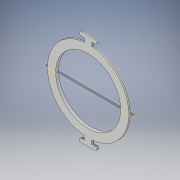
# Autodesk Inventor part: Baseplate_mitte
Saved by Autodesk Inventor 2018 (Build 220112000, 112)
## iProperties
Created: 2020-01-15
Part Number: Baseplate_mitte
Material: Generisch
Document SubType Name: Modeling
Designer: maxse
Density: 1 g/cm^3
Appearance: Vorgabe
Author: maxse
Autodesk Inventor part; units mm, degrees
(part 1 of 3)
ref_plane "YZ Plane" through (0, 0, 0) normal (1, 0, 0) x (0, 1, 0)
ref_plane "XZ Plane" through (0, 0, 0) normal (0, 1, 0) x (-1, 0, 0)
ref_plane "XY Plane" through (0, 0, 0) normal (0, 0, 1) x (1, 0, 0)
sketch "Skizze1" plane through (0, 0, 0) normal (0, 1, 0) x (-1, 0, 0)
  circle A0 centre (0, 0) radius 55
  circle A1 centre (0, 0) radius 44
  line L0 (-9.5, -65) -> (9.5, -65)
  line L1 (-9.5, -60) -> (-5, -60)
  line L2 (-5, -60) -> (-5, -54.7723)
  line L3 (5, -54.7723) -> (5, -60)
  line L4 (5, -60) -> (9.5, -60)
  arc A2 (9.5, -65) -> (9.5, -60) centre (9.5, -62.5) ccw
  arc A3 (-9.5, -60) -> (-9.5, -65) centre (-9.5, -62.5) ccw
  dimension "d0" = 110
  dimension "d1" = 88
  dimension "d2" = 10
  dimension "d3" = 2.5
  dimension "d4" = 2.5
  dimension "d5" = 5
  dimension "d6" = 5
  dimension "d7" = 24
  dimension "d8" = 60
  dimension "d9" = 4.5
  constraints: 10 end point, 6 point on circle, 4 centre point, 2 coincident, 2 horizontal, 2 point on line, 1 parallel, 1 perpendicular
  measures "d0" diameter of A0
  measures "d1" diameter of A1
  measures "d2" distance between parallel lines of L3 L2
  measures "d3" radius of A2
  measures "d4" radius of A3
  measures "d5" distance between parallel lines of L1 L0
  measures "d6" distance from line of point (0, 0) L2
  measures "d8" distance from line of A0.centre L4
  measures "d9" distance from line of L3 A2.centre
extrude "Extrusion1" add sketch "Skizze1" along normal blind 4
mirror "Spiegeln1" about plane through (0, 0, 0) normal (0, 0, 1) of "Extrusion1"
sketch "Skizze2" plane through (0, 4, 0) normal (0, 1, 0) x (1, 0, 0)
  circle A0 centre (0, 0) radius 45 projected
  line L0 (42.831, 23.1383) -> (42.0944, 24.3949)
  line L1 (42.0944, 24.3949) -> (40.8378, 23.6583)
  line L2 (40.8378, 23.6583) -> (40.5946, 24.0731)
  line L3 (40.5946, 24.0731) -> (41.8512, 24.8097)
  line L4 (41.8512, 24.8097) -> (41.1146, 26.0663)
  line L5 (41.1146, 26.0663) -> (41.5144, 26.3007)
  line L6 (41.5144, 26.3007) -> (42.251, 25.0441)
  line L7 (42.251, 25.0441) -> (43.5076, 25.7807)
  line L8 (43.5076, 25.7807) -> (43.7508, 25.3659)
  line L9 (43.7508, 25.3659) -> (42.4942, 24.6293)
  line L10 (42.4942, 24.6293) -> (43.2308, 23.3727)
  line L11 (43.2308, 23.3727) -> (42.831, 23.1383)
  line L12 (44.766, 19.128) -> (44.1473, 20.4466)
  line L13 (44.1473, 20.4466) -> (42.8287, 19.8279)
  line L14 (42.8287, 19.8279) -> (42.6244, 20.2632)
  line L15 (42.6244, 20.2632) -> (43.943, 20.8819)
  line L16 (43.943, 20.8819) -> (43.3243, 22.2006)
  line L17 (43.3243, 22.2006) -> (43.7439, 22.3974)
  line L18 (43.7439, 22.3974) -> (44.3626, 21.0788)
  line L19 (44.3626, 21.0788) -> (45.6812, 21.6975)
  line L20 (45.6812, 21.6975) -> (45.8855, 21.2622)
  line L21 (45.8855, 21.2622) -> (44.5669, 20.6435)
  line L22 (44.5669, 20.6435) -> (45.1856, 19.3248)
  line L23 (45.1856, 19.3248) -> (44.766, 19.128)
  line L24 (46.3265, 14.9576) -> (45.8309, 16.3272)
  line L25 (45.8309, 16.3272) -> (44.4612, 15.8316)
  line L26 (44.4612, 15.8316) -> (44.2976, 16.2838)
  line L27 (44.2976, 16.2838) -> (45.6672, 16.7794)
  line L28 (45.6672, 16.7794) -> (45.1716, 18.1491)
  line L29 (45.1716, 18.1491) -> (45.6074, 18.3068)
  line L30 (45.6074, 18.3068) -> (46.103, 16.9371)
  line L31 (46.103, 16.9371) -> (47.4727, 17.4328)
  line L32 (47.4727, 17.4328) -> (47.6363, 16.9806)
  line L33 (47.6363, 16.9806) -> (46.2667, 16.4849)
  line L34 (46.2667, 16.4849) -> (46.7623, 15.1153)
  line L35 (46.7623, 15.1153) -> (46.3265, 14.9576)
  line L36 (48.9055, 8.9669) -> (48.7236, 9.7939)
  line L37 (48.7236, 9.7939) -> (47.6091, 9.8164)
  line L38 (47.6091, 9.8164) -> (47.7745, 9.0643)
  line L39 (47.7745, 9.0643) -> (47.3933, 8.9805)
  line L40 (47.3933, 8.9805) -> (47.2062, 9.8313)
  line L41 (47.2062, 9.8313) -> (45.9534, 9.8662)
  line L42 (45.9534, 9.8662) -> (45.8733, 10.2304)
  line L43 (45.8733, 10.2304) -> (47.1262, 10.1954)
  line L44 (47.1262, 10.1954) -> (46.957, 10.9646)
  line L45 (46.957, 10.9646) -> (45.7042, 10.9995)
  line L46 (45.7042, 10.9995) -> (45.6241, 11.3637)
  line L47 (45.6241, 11.3637) -> (46.877, 11.3287)
  line L48 (46.877, 11.3287) -> (46.7168, 12.0571)
  line L49 (46.7168, 12.0571) -> (47.098, 12.1409)
  line L50 (47.098, 12.1409) -> (47.2798, 11.3139)
  line L51 (47.2798, 11.3139) -> (48.3944, 11.2913)
  line L52 (48.3944, 11.2913) -> (48.229, 12.0434)
  line L53 (48.229, 12.0434) -> (48.6102, 12.1273)
  line L54 (48.6102, 12.1273) -> (48.7973, 11.2764)
  line L55 (48.7973, 11.2764) -> (50.0535, 11.2422)
  line L56 (50.0535, 11.2422) -> (50.1336, 10.8781)
  line L57 (50.1336, 10.8781) -> (48.8773, 10.9123)
  line L58 (48.8773, 10.9123) -> (49.0464, 10.1431)
  line L59 (49.0464, 10.1431) -> (50.3027, 10.1089)
  line L60 (50.3027, 10.1089) -> (50.3828, 9.7448)
  line L61 (50.3828, 9.7448) -> (49.1265, 9.779)
  line L62 (49.1265, 9.779) -> (49.2866, 9.0507)
  line L63 (49.2866, 9.0507) -> (48.9055, 8.9669)
  line L64 (48.6526, 10.1493) -> (48.4813, 10.9287)
  line L65 (48.4813, 10.9287) -> (47.3516, 10.955)
  line L66 (47.3516, 10.955) -> (47.523, 10.1757)
  line L67 (47.523, 10.1757) -> (48.6526, 10.1493)
  spline S0 degree 2 poles (48.4497, 5.1486) (47.6487, 5.0391) (46.5984, 5.6727) (46.5186, 6.2562) knots 0 0 0 1 2 2 2
  spline S1 degree 2 poles (46.5186, 6.2562) (46.486, 6.4944) (46.5464, 6.8755) (46.6344, 7.0809) knots 0 0 0 1 2 2 2
  line L68 (46.6344, 7.0809) -> (45.2948, 6.8977)
  line L69 (45.2948, 6.8977) -> (45.2212, 7.4363)
  line L70 (45.2212, 7.4363) -> (49.5955, 8.0345)
  line L71 (49.5955, 8.0345) -> (49.6691, 7.496)
  line L72 (49.6691, 7.496) -> (49.3342, 7.4502)
  spline S2 degree 2 poles (49.3342, 7.4502) (49.5446, 7.2749) (49.8533, 6.8177) (49.8925, 6.5312) knots 0 0 0 1 2 2 2
  spline S3 degree 2 poles (49.8925, 6.5312) (49.9676, 5.9822) (49.1816, 5.2487) (48.4497, 5.1486) knots 0 0 0 1 2 2 2
  spline S4 degree 2 poles (48.3115, 5.696) (48.8605, 5.771) (49.417, 6.2024) (49.3636, 6.5925) knots 0 0 0 1 2 2 2
  spline S5 degree 2 poles (49.3636, 6.5925) (49.3324, 6.8204) (49.0702, 7.2206) (48.8854, 7.3888) knots 0 0 0 1 2 2 2
  line L73 (48.8854, 7.3888) -> (47.0694, 7.1404)
  spline S6 degree 2 poles (47.0694, 7.1404) (46.9981, 6.9161) (46.9632, 6.6054) (46.9897, 6.412) knots 0 0 0 1 2 2 2
  spline S7 degree 2 poles (46.9897, 6.412) (47.0468, 5.9943) (47.7246, 5.6157) (48.3115, 5.696) knots 0 0 0 1 2 2 2
  line L74 (46.8467, 3.8024) -> (46.7996, 4.344)
  line L75 (46.7996, 4.344) -> (50.0142, 4.6236)
  line L76 (50.0142, 4.6236) -> (50.0613, 4.0821)
  line L77 (50.0613, 4.0821) -> (46.8467, 3.8024)
  line L78 (50.5993, 4.0904) -> (50.5458, 4.7048)
  line L79 (50.5458, 4.7048) -> (51.1082, 4.7538)
  line L80 (51.1082, 4.7538) -> (51.1616, 4.1393)
  line L81 (51.1616, 4.1393) -> (50.5993, 4.0904)
  line L82 (47.0217, -0.6477) -> (48.8891, -0.6111)
  spline S8 degree 2 poles (48.8891, -0.6111) (49.1121, -0.6067) (49.4912, -0.5644) (49.5946, -0.5066) knots 0 0 0 1 2 2 2
  spline S9 degree 2 poles (49.5946, -0.5066) (49.7085, -0.4486) (49.8158, -0.2339) (49.8122, -0.0493) knots 0 0 0 1 2 2 2
  spline S10 degree 2 poles (49.8122, -0.0493) (49.8089, 0.118) (49.5958, 0.4972) (49.3968, 0.6954) knots 0 0 0 1 2 2 2
  spline S11 degree 2 poles (49.3968, 0.6954) (49.348, 0.691) (49.2123, 0.6813) (49.1217, 0.6796) knots 0 0 0 1 2 2 2
  line L83 (49.1217, 0.6796) -> (46.9965, 0.6379)
  line L84 (46.9965, 0.6379) -> (46.9859, 1.1814)
  line L85 (46.9859, 1.1814) -> (48.8533, 1.218)
  spline S12 degree 2 poles (48.8533, 1.218) (49.0762, 1.2224) (49.4553, 1.2647) (49.5587, 1.3225) knots 0 0 0 1 2 2 2
  spline S13 degree 2 poles (49.5587, 1.3225) (49.6726, 1.3805) (49.7799, 1.5952) (49.7763, 1.7798) knots 0 0 0 1 2 2 2
  spline S14 degree 2 poles (49.7763, 1.7798) (49.7729, 1.954) (49.5458, 2.3364) (49.3715, 2.5142) knots 0 0 0 1 2 2 2
  line L86 (49.3715, 2.5142) -> (46.9606, 2.4669)
  line L87 (46.9606, 2.4669) -> (46.95, 3.0104)
  line L88 (46.95, 3.0104) -> (50.1761, 3.0737)
  line L89 (50.1761, 3.0737) -> (50.1868, 2.5302)
  line L90 (50.1868, 2.5302) -> (49.8314, 2.5233)
  spline S15 degree 2 poles (49.8314, 2.5233) (50.0481, 2.3149) (50.2897, 1.9014) (50.2946, 1.6506) knots 0 0 0 1 2 2 2
  spline S16 degree 2 poles (50.2946, 1.6506) (50.3002, 1.3649) (50.0476, 0.9173) (49.7538, 0.7965) knots 0 0 0 1 2 2 2
  spline S17 degree 2 poles (49.7538, 0.7965) (50.0338, 0.5546) (50.3252, 0.0933) (50.3305, -0.1785) knots 0 0 0 1 2 2 2
  spline S18 degree 2 poles (50.3305, -0.1785) (50.3346, -0.3875) (50.2124, -0.7315) (50.0686, -0.8598) knots 0 0 0 1 2 2 2
  spline S19 degree 2 poles (50.0686, -0.8598) (49.9248, -0.9916) (49.4886, -1.143) (49.1576, -1.1495) knots 0 0 0 1 2 2 2
  line L91 (49.1576, -1.1495) -> (47.0324, -1.1912)
  line L92 (47.0324, -1.1912) -> (47.0217, -0.6477)
  spline S20 degree 2 poles (48.4889, -4.7653) (47.6823, -4.7105) (46.782, -3.8773) (46.822, -3.2898) knots 0 0 0 1 2 2 2
  spline S21 degree 2 poles (46.822, -3.2898) (46.8383, -3.0499) (46.9746, -2.689) (47.1023, -2.5056) knots 0 0 0 1 2 2 2
  line L93 (47.1023, -2.5056) -> (45.7534, -2.4138)
  line L94 (45.7534, -2.4138) -> (45.7903, -1.8715)
  line L95 (45.7903, -1.8715) -> (50.1951, -2.1711)
  line L96 (50.1951, -2.1711) -> (50.1582, -2.7134)
  line L97 (50.1582, -2.7134) -> (49.821, -2.6905)
  spline S22 degree 2 poles (49.821, -2.6905) (49.9916, -2.9047) (50.2013, -3.4149) (50.1817, -3.7035) knots 0 0 0 1 2 2 2
  spline S23 degree 2 poles (50.1817, -3.7035) (50.1441, -4.2562) (49.2259, -4.8155) (48.4889, -4.7653) knots 0 0 0 1 2 2 2
  spline S24 degree 2 poles (48.4644, -4.2013) (49.0171, -4.2389) (49.6494, -3.9292) (49.6762, -3.5363) knots 0 0 0 1 2 2 2
  spline S25 degree 2 poles (49.6762, -3.5363) (49.6918, -3.3069) (49.516, -2.8618) (49.3691, -2.6598) knots 0 0 0 1 2 2 2
  line L98 (49.3691, -2.6598) -> (47.5404, -2.5354)
  spline S26 degree 2 poles (47.5404, -2.5354) (47.4251, -2.7406) (47.3281, -3.0378) (47.3148, -3.2325) knots 0 0 0 1 2 2 2
  spline S27 degree 2 poles (47.3148, -3.2325) (47.2862, -3.6532) (47.8734, -4.1611) (48.4644, -4.2013) knots 0 0 0 1 2 2 2
  line L99 (49.5822, -8.1516) -> (45.4386, -5.842)
  line L100 (45.4386, -5.842) -> (45.5163, -5.2653)
  line L101 (45.5163, -5.2653) -> (46.7721, -6.0183)
  line L102 (46.7721, -6.0183) -> (49.9709, -5.2681)
  line L103 (49.9709, -5.2681) -> (49.8927, -5.8482)
  line L104 (49.8927, -5.8482) -> (47.4059, -6.4026)
  line L105 (47.4059, -6.4026) -> (49.6576, -7.5922)
  line L106 (49.6576, -7.5922) -> (49.5822, -8.1516)
  spline S28 degree 2 poles (47.3643, -11.0433) (46.5651, -10.8818) (45.8495, -9.9373) (45.9793, -9.2951) knots 0 0 0 1 2 2 2
  spline S29 degree 2 poles (45.9793, -9.2951) (46.1125, -8.6359) (47.1633, -8.0627) (47.9353, -8.2187) knots 0 0 0 1 2 2 2
  spline S30 degree 2 poles (47.9353, -8.2187) (48.7277, -8.3789) (49.4481, -9.335) (49.3196, -9.9703) knots 0 0 0 1 2 2 2
  spline S31 degree 2 poles (49.3196, -9.9703) (49.1899, -10.6124) (48.1602, -11.2042) (47.3643, -11.0433) knots 0 0 0 1 2 2 2
  spline S32 degree 2 poles (47.4755, -10.4934) (48.0903, -10.6177) (48.7784, -10.2911) (48.862, -9.8778) knots 0 0 0 1 2 2 2
  spline S33 degree 2 poles (48.862, -9.8778) (48.9455, -9.4645) (48.4389, -8.8929) (47.8241, -8.7686) knots 0 0 0 1 2 2 2
  spline S34 degree 2 poles (47.8241, -8.7686) (47.2264, -8.6478) (46.5205, -8.9744) (46.4369, -9.3877) knots 0 0 0 1 2 2 2
  spline S35 degree 2 poles (46.4369, -9.3877) (46.3541, -9.7975) (46.8675, -10.3706) (47.4755, -10.4934) knots 0 0 0 1 2 2 2
  line L107 (44.9816, -13.6832) -> (45.1259, -13.1591)
  line L108 (45.1259, -13.1591) -> (45.4686, -13.2534)
  spline S36 degree 2 poles (45.4686, -13.2534) (45.3235, -12.9532) (45.2244, -12.4597) (45.2984, -12.191) knots 0 0 0 1 2 2 2
  spline S37 degree 2 poles (45.2984, -12.191) (45.3539, -11.9894) (45.5872, -11.6669) (45.7678, -11.5756) knots 0 0 0 1 2 2 2
  spline S38 degree 2 poles (45.7678, -11.5756) (45.9492, -11.481) (46.43, -11.4543) (46.7458, -11.5413) knots 0 0 0 1 2 2 2
  line L109 (46.7458, -11.5413) -> (48.765, -12.0971)
  line L110 (48.765, -12.0971) -> (48.6207, -12.6212)
  line L111 (48.6207, -12.6212) -> (46.8468, -12.1329)
  spline S39 degree 2 poles (46.8468, -12.1329) (46.5982, -12.0645) (46.2621, -12.0117) (46.1236, -12.0422) knots 0 0 0 1 2 2 2
  spline S40 degree 2 poles (46.1236, -12.0422) (45.9851, -12.0728) (45.8141, -12.2606) (45.7577, -12.4656) knots 0 0 0 1 2 2 2
  spline S41 degree 2 poles (45.7577, -12.4656) (45.705, -12.6571) (45.8041, -13.1506) (45.912, -13.3755) knots 0 0 0 1 2 2 2
  line L112 (45.912, -13.3755) -> (48.2369, -14.0154)
  line L113 (48.2369, -14.0154) -> (48.0926, -14.5395)
  line L114 (48.0926, -14.5395) -> (44.9816, -13.6832)
  line L115 (46.6915, -16.8993) -> (46.7005, -16.8729)
  spline S42 degree 2 poles (46.7005, -16.8729) (46.7371, -16.8191) (46.7873, -16.6926) (46.8174, -16.6035) knots 0 0 0 1 2 2 2
  spline S43 degree 2 poles (46.8174, -16.6035) (46.8878, -16.3955) (46.8448, -15.9248) (46.7291, -15.6796) knots 0 0 0 1 2 2 2
  line L116 (46.7291, -15.6796) -> (44.5606, -14.9457)
  line L117 (44.5606, -14.9457) -> (44.7348, -14.4308)
  line L118 (44.7348, -14.4308) -> (47.7913, -15.4652)
  line L119 (47.7913, -15.4652) -> (47.617, -15.9801)
  line L120 (47.617, -15.9801) -> (47.1615, -15.826)
  spline S44 degree 2 poles (47.1615, -15.826) (47.3174, -16.1914) (47.3802, -16.6799) (47.3131, -16.8779) knots 0 0 0 1 2 2 2
  spline S45 degree 2 poles (47.3131, -16.8779) (47.2863, -16.9571) (47.2529, -17.0341) (47.2262, -17.0803) knots 0 0 0 1 2 2 2
  line L121 (47.2262, -17.0803) -> (46.6915, -16.8993)
  spline S46 degree 2 poles (44.6095, -19.5926) (43.8599, -19.2899) (43.263, -18.2183) (43.4835, -17.6722) knots 0 0 0 1 2 2 2
  spline S47 degree 2 poles (43.4835, -17.6722) (43.5735, -17.4493) (43.8152, -17.1485) (43.9936, -17.0139) knots 0 0 0 1 2 2 2
  line L122 (43.9936, -17.0139) -> (42.7399, -16.5076)
  line L123 (42.7399, -16.5076) -> (42.9435, -16.0036)
  line L124 (42.9435, -16.0036) -> (47.0373, -17.6567)
  line L125 (47.0373, -17.6567) -> (46.8337, -18.1608)
  line L126 (46.8337, -18.1608) -> (46.5203, -18.0342)
  spline S48 degree 2 poles (46.5203, -18.0342) (46.6159, -18.2908) (46.6568, -18.8409) (46.5485, -19.1091) knots 0 0 0 1 2 2 2
  spline S49 degree 2 poles (46.5485, -19.1091) (46.341, -19.6228) (45.2945, -19.8692) (44.6095, -19.5926) knots 0 0 0 1 2 2 2
  spline S50 degree 2 poles (44.7614, -19.0489) (45.2752, -19.2563) (45.9724, -19.1583) (46.1199, -18.7932) knots 0 0 0 1 2 2 2
  spline S51 degree 2 poles (46.1199, -18.7932) (46.206, -18.58) (46.1771, -18.1023) (46.1003, -17.8646) knots 0 0 0 1 2 2 2
  line L127 (46.1003, -17.8646) -> (44.4007, -17.1783)
  spline S52 degree 2 poles (44.4007, -17.1783) (44.2274, -17.3375) (44.0428, -17.5899) (43.9697, -17.7709) knots 0 0 0 1 2 2 2
  spline S53 degree 2 poles (43.9697, -17.7709) (43.8119, -18.1618) (44.2122, -18.8271) (44.7614, -19.0489) knots 0 0 0 1 2 2 2
  line L128 (44.4466, -22.1401) -> (44.4585, -22.1149)
  spline S54 degree 2 poles (44.4585, -22.1149) (44.501, -22.0657) (44.5654, -21.9457) (44.6056, -21.8607) knots 0 0 0 1 2 2 2
  spline S55 degree 2 poles (44.6056, -21.8607) (44.6993, -21.6622) (44.7105, -21.1896) (44.6237, -20.9328) knots 0 0 0 1 2 2 2
  line L129 (44.6237, -20.9328) -> (42.5536, -19.9551)
  line L130 (42.5536, -19.9551) -> (42.7858, -19.4636)
  line L131 (42.7858, -19.4636) -> (45.7035, -20.8416)
  line L132 (45.7035, -20.8416) -> (45.4713, -21.3331)
  line L133 (45.4713, -21.3331) -> (45.0365, -21.1277)
  spline S56 degree 2 poles (45.0365, -21.1277) (45.1495, -21.5087) (45.1558, -22.0011) (45.0665, -22.1901) knots 0 0 0 1 2 2 2
  spline S57 degree 2 poles (45.0665, -22.1901) (45.0308, -22.2658) (44.9888, -22.3384) (44.957, -22.3812) knots 0 0 0 1 2 2 2
  line L134 (44.957, -22.3812) -> (44.4466, -22.1401)
  line L135 (41.6005, -21.8741) -> (41.8507, -21.3915)
  line L136 (41.8507, -21.3915) -> (44.7153, -22.8766)
  line L137 (44.7153, -22.8766) -> (44.4651, -23.3592)
  line L138 (44.4651, -23.3592) -> (41.6005, -21.8741)
  line L139 (44.9239, -23.6403) -> (45.2078, -23.0927)
  line L140 (45.2078, -23.0927) -> (45.7089, -23.3525)
  line L141 (45.7089, -23.3525) -> (45.425, -23.9001)
  line L142 (45.425, -23.9001) -> (44.9239, -23.6403)
  line L143 (39.9616, -24.7731) -> (40.2353, -24.3035)
  line L144 (40.2353, -24.3035) -> (41.8249, -25.23)
  spline S58 degree 2 poles (41.8249, -25.23) (42.0176, -25.3423) (42.3698, -25.4992) (42.5007, -25.5029) knots 0 0 0 1 2 2 2
  spline S59 degree 2 poles (42.5007, -25.5029) (42.6394, -25.5071) (42.8611, -25.3621) (42.9629, -25.1875) knots 0 0 0 1 2 2 2
  spline S60 degree 2 poles (42.9629, -25.1875) (43.0646, -25.0129) (43.0938, -24.5338) (43.0468, -24.2684) knots 0 0 0 1 2 2 2
  line L145 (43.0468, -24.2684) -> (40.9636, -23.0541)
  line L146 (40.9636, -23.0541) -> (41.2373, -22.5845)
  line L147 (41.2373, -22.5845) -> (44.025, -24.2094)
  line L148 (44.025, -24.2094) -> (43.7513, -24.679)
  line L149 (43.7513, -24.679) -> (43.4412, -24.4983)
  spline S61 degree 2 poles (43.4412, -24.4983) (43.508, -24.8196) (43.4698, -25.3418) (43.3365, -25.5706) knots 0 0 0 1 2 2 2
  spline S62 degree 2 poles (43.3365, -25.5706) (43.0978, -25.98) (42.2857, -26.1278) (41.7709, -25.8277) knots 0 0 0 1 2 2 2
  line L150 (41.7709, -25.8277) -> (39.9616, -24.7731)
  spline S63 degree 2 poles (38.9527, -26.1904) (39.1967, -25.8212) (39.8929, -25.6839) (40.3494, -25.9855) knots 0 0 0 1 2 2 2
  line L151 (40.3494, -25.9855) -> (41.8409, -26.9709)
  line L152 (41.8409, -26.9709) -> (42.0426, -26.6656)
  line L153 (42.0426, -26.6656) -> (42.4176, -26.9134)
  line L154 (42.4176, -26.9134) -> (42.2159, -27.2187)
  line L155 (42.2159, -27.2187) -> (42.9893, -27.7296)
  line L156 (42.9893, -27.7296) -> (42.6896, -28.1832)
  line L157 (42.6896, -28.1832) -> (41.9163, -27.6722)
  line L158 (41.9163, -27.6722) -> (41.365, -28.5066)
  line L159 (41.365, -28.5066) -> (40.9899, -28.2589)
  line L160 (40.9899, -28.2589) -> (41.5412, -27.4244)
  line L161 (41.5412, -27.4244) -> (40.2591, -26.5774)
  spline S64 degree 2 poles (40.2591, -26.5774) (40.0555, -26.4429) (39.8221, -26.3095) (39.6935, -26.2956) knots 0 0 0 1 2 2 2
  spline S65 degree 2 poles (39.6935, -26.2956) (39.5823, -26.2806) (39.3769, -26.408) (39.2732, -26.565) knots 0 0 0 1 2 2 2
  spline S66 degree 2 poles (39.2732, -26.565) (39.2002, -26.6755) (39.1307, -26.9261) (39.1203, -26.9861) knots 0 0 0 1 2 2 2
  line L162 (39.1203, -26.9861) -> (39.1031, -27.0122)
  line L163 (39.1031, -27.0122) -> (38.696, -26.7433)
  spline S67 degree 2 poles (38.696, -26.7433) (38.7456, -26.5923) (38.8778, -26.3038) (38.9527, -26.1904) knots 0 0 0 1 2 2 2
  line L164 (36.4432, -32.2764) -> (37.3703, -31.153)
  line L165 (37.3703, -31.153) -> (36.2468, -30.2259)
  line L166 (36.2468, -30.2259) -> (36.5529, -29.855)
  line L167 (36.5529, -29.855) -> (37.6763, -30.7821)
  line L168 (37.6763, -30.7821) -> (38.6034, -29.6587)
  line L169 (38.6034, -29.6587) -> (38.9609, -29.9537)
  line L170 (38.9609, -29.9537) -> (38.0338, -31.0771)
  line L171 (38.0338, -31.0771) -> (39.1572, -32.0042)
  line L172 (39.1572, -32.0042) -> (38.8511, -32.3751)
  line L173 (38.8511, -32.3751) -> (37.7277, -31.448)
  line L174 (37.7277, -31.448) -> (36.8006, -32.5714)
  line L175 (36.8006, -32.5714) -> (36.4432, -32.2764)
  line L176 (33.3416, -35.4713) -> (34.3674, -34.4373)
  line L177 (34.3674, -34.4373) -> (33.3334, -33.4114)
  line L178 (33.3334, -33.4114) -> (33.6721, -33.0701)
  line L179 (33.6721, -33.0701) -> (34.7061, -34.0959)
  line L180 (34.7061, -34.0959) -> (35.732, -33.0619)
  line L181 (35.732, -33.0619) -> (36.061, -33.3883)
  line L182 (36.061, -33.3883) -> (35.0351, -34.4223)
  line L183 (35.0351, -34.4223) -> (36.0691, -35.4482)
  line L184 (36.0691, -35.4482) -> (35.7304, -35.7896)
  line L185 (35.7304, -35.7896) -> (34.6964, -34.7637)
  line L186 (34.6964, -34.7637) -> (33.6706, -35.7977)
  line L187 (33.6706, -35.7977) -> (33.3416, -35.4713)
  line L188 (29.961, -38.3694) -> (31.077, -37.4335)
  line L189 (31.077, -37.4335) -> (30.1411, -36.3174)
  line L190 (30.1411, -36.3174) -> (30.5095, -36.0084)
  line L191 (30.5095, -36.0084) -> (31.4455, -37.1245)
  line L192 (31.4455, -37.1245) -> (32.5616, -36.1885)
  line L193 (32.5616, -36.1885) -> (32.8594, -36.5436)
  line L194 (32.8594, -36.5436) -> (31.7433, -37.4796)
  line L195 (31.7433, -37.4796) -> (32.6793, -38.5956)
  line L196 (32.6793, -38.5956) -> (32.3108, -38.9046)
  line L197 (32.3108, -38.9046) -> (31.3749, -37.7886)
  line L198 (31.3749, -37.7886) -> (30.2588, -38.7245)
  line L199 (30.2588, -38.7245) -> (29.961, -38.3694)
  line L200 (23.5821, -40.6975) -> (24.065, -40.3918)
  line L201 (24.065, -40.3918) -> (26.0462, -43.5215)
  line L202 (26.0462, -43.5215) -> (25.6467, -40.7927)
  line L203 (25.6467, -40.7927) -> (25.9411, -40.6063)
  line L204 (25.9411, -40.6063) -> (28.2279, -42.1404)
  line L205 (28.2279, -42.1404) -> (26.2466, -39.0107)
  line L206 (26.2466, -39.0107) -> (26.6971, -38.7255)
  line L207 (26.6971, -38.7255) -> (28.9971, -42.3587)
  line L208 (28.9971, -42.3587) -> (28.3376, -42.7762)
  line L209 (28.3376, -42.7762) -> (26.1503, -41.3276)
  line L210 (26.1503, -41.3276) -> (26.5534, -43.9057)
  line L211 (26.5534, -43.9057) -> (25.8821, -44.3306)
  line L212 (25.8821, -44.3306) -> (23.5821, -40.6975)
  spline S68 degree 2 poles (21.5761, -41.6732) (22.2613, -41.314) (23.4172, -41.6877) (23.7893, -42.3976) knots 0 0 0 1 2 2 2
  spline S69 degree 2 poles (23.7893, -42.3976) (24.1549, -43.0951) (23.8571, -44.3056) (23.2676, -44.6146) knots 0 0 0 1 2 2 2
  spline S70 degree 2 poles (23.2676, -44.6146) (23.0022, -44.7538) (22.5108, -44.8146) (22.2738, -44.7303) knots 0 0 0 1 2 2 2
  spline S71 degree 2 poles (22.2738, -44.7303) (22.0338, -44.6477) (21.6227, -44.2612) (21.4431, -43.9186) knots 0 0 0 1 2 2 2
  line L213 (21.4431, -43.9186) -> (21.3056, -43.6563)
  line L214 (21.3056, -43.6563) -> (23.2839, -42.6193)
  spline S72 degree 2 poles (23.2839, -42.6193) (23.0234, -42.1224) (22.2468, -41.8567) (21.8023, -42.0897) knots 0 0 0 1 2 2 2
  spline S73 degree 2 poles (21.8023, -42.0897) (21.6449, -42.1722) (21.3766, -42.4033) (21.2823, -42.5236) knots 0 0 0 1 2 2 2
  spline S74 degree 2 poles (21.2823, -42.5236) (21.185, -42.6533) (21.0626, -42.8551) (21.0299, -42.9353) knots 0 0 0 1 2 2 2
  line L215 (21.0299, -42.9353) -> (21.0021, -42.9498)
  line L216 (21.0021, -42.9498) -> (20.7271, -42.4252)
  spline S75 degree 2 poles (20.7271, -42.4252) (20.7926, -42.3475) (20.9939, -42.1161) (21.0781, -42.0366) knots 0 0 0 1 2 2 2
  spline S76 degree 2 poles (21.0781, -42.0366) (21.1959, -41.9236) (21.4033, -41.7638) (21.5761, -41.6732) knots 0 0 0 1 2 2 2
  spline S77 degree 2 poles (21.9672, -43.7777) (22.0753, -43.9688) (22.3044, -44.2107) (22.4317, -44.2659) knots 0 0 0 1 2 2 2
  spline S78 degree 2 poles (22.4317, -44.2659) (22.5716, -44.3303) (22.8938, -44.307) (23.0883, -44.205) knots 0 0 0 1 2 2 2
  spline S79 degree 2 poles (23.0883, -44.205) (23.2796, -44.1047) (23.4883, -43.8498) (23.5411, -43.6804) knots 0 0 0 1 2 2 2
  spline S80 degree 2 poles (23.5411, -43.6804) (23.5893, -43.5096) (23.5564, -43.1767) (23.4764, -42.9865) knots 0 0 0 1 2 2 2
  line L217 (23.4764, -42.9865) -> (21.9672, -43.7777)
  line L218 (16.7233, -43.9522) -> (17.4454, -45.6747)
  spline S81 degree 2 poles (17.4454, -45.6747) (17.5317, -45.8804) (17.7106, -46.2172) (17.8025, -46.292) knots 0 0 0 1 2 2 2
  spline S82 degree 2 poles (17.8025, -46.292) (17.8984, -46.3765) (18.1375, -46.3972) (18.3078, -46.3258) knots 0 0 0 1 2 2 2
  spline S83 degree 2 poles (18.3078, -46.3258) (18.4621, -46.2611) (18.7361, -45.9233) (18.847, -45.6652) knots 0 0 0 1 2 2 2
  spline S84 degree 2 poles (18.847, -45.6652) (18.825, -45.6216) (18.766, -45.4989) (18.731, -45.4154) knots 0 0 0 1 2 2 2
  line L219 (18.731, -45.4154) -> (17.9092, -43.4551)
  line L220 (17.9092, -43.4551) -> (18.4105, -43.2449)
  line L221 (18.4105, -43.2449) -> (19.1326, -44.9674)
  spline S85 degree 2 poles (19.1326, -44.9674) (19.2188, -45.1731) (19.3978, -45.5099) (19.4896, -45.5847) knots 0 0 0 1 2 2 2
  spline S86 degree 2 poles (19.4896, -45.5847) (19.5855, -45.6692) (19.8247, -45.6899) (19.995, -45.6185) knots 0 0 0 1 2 2 2
  spline S87 degree 2 poles (19.995, -45.6185) (20.1557, -45.5511) (20.4275, -45.1991) (20.5286, -44.9716) knots 0 0 0 1 2 2 2
  line L222 (20.5286, -44.9716) -> (19.5963, -42.7478)
  line L223 (19.5963, -42.7478) -> (20.0977, -42.5376)
  line L224 (20.0977, -42.5376) -> (21.3452, -45.5134)
  line L225 (21.3452, -45.5134) -> (20.8438, -45.7236)
  line L226 (20.8438, -45.7236) -> (20.7064, -45.3958)
  spline S88 degree 2 poles (20.7064, -45.3958) (20.5926, -45.674) (20.2972, -46.051) (20.0658, -46.148) knots 0 0 0 1 2 2 2
  spline S89 degree 2 poles (20.0658, -46.148) (19.8023, -46.2585) (19.2931, -46.1885) (19.0726, -45.9598) knots 0 0 0 1 2 2 2
  spline S90 degree 2 poles (19.0726, -45.9598) (18.9508, -46.3094) (18.6293, -46.7502) (18.3787, -46.8553) knots 0 0 0 1 2 2 2
  spline S91 degree 2 poles (18.3787, -46.8553) (18.1858, -46.9361) (17.8211, -46.9492) (17.6488, -46.8628) knots 0 0 0 1 2 2 2
  spline S92 degree 2 poles (17.6488, -46.8628) (17.4733, -46.7776) (17.1718, -46.428) (17.0438, -46.1227) knots 0 0 0 1 2 2 2
  line L227 (17.0438, -46.1227) -> (16.222, -44.1623)
  line L228 (16.222, -44.1623) -> (16.7233, -43.9522)
  spline S93 degree 2 poles (13.4254, -46.8001) (13.1845, -46.0466) (13.6208, -44.8938) (14.1717, -44.7176) knots 0 0 0 1 2 2 2
  spline S94 degree 2 poles (14.1717, -44.7176) (14.4207, -44.6381) (14.8151, -44.6473) (15.0216, -44.6984) knots 0 0 0 1 2 2 2
  line L229 (15.0216, -44.6984) -> (15.0092, -44.545)
  line L230 (15.0092, -44.545) -> (15.4938, -44.3901)
  line L231 (15.4938, -44.3901) -> (16.8615, -48.6684)
  line L232 (16.8615, -48.6684) -> (16.3438, -48.834)
  line L233 (16.3438, -48.834) -> (15.8557, -47.3072)
  spline S95 degree 2 poles (15.8557, -47.3072) (15.7161, -47.5457) (15.3356, -47.9234) (15.0469, -48.0157) knots 0 0 0 1 2 2 2
  spline S96 degree 2 poles (15.0469, -48.0157) (14.5258, -48.1823) (13.662, -47.5402) (13.4254, -46.8001) knots 0 0 0 1 2 2 2
  spline S97 degree 2 poles (13.947, -46.5894) (14.1231, -47.1404) (14.6409, -47.6041) (15.0126, -47.4852) knots 0 0 0 1 2 2 2
  spline S98 degree 2 poles (15.0126, -47.4852) (15.2217, -47.4184) (15.5895, -47.0813) (15.7166, -46.8724) knots 0 0 0 1 2 2 2
  line L234 (15.7166, -46.8724) -> (15.1532, -45.1099)
  spline S99 degree 2 poles (15.1532, -45.1099) (14.9266, -45.0763) (14.5991, -45.0932) (14.4199, -45.1505) knots 0 0 0 1 2 2 2
  spline S100 degree 2 poles (14.4199, -45.1505) (14.0249, -45.2768) (13.7528, -45.982) (13.947, -46.5894) knots 0 0 0 1 2 2 2
  line L235 (11.3723, -48.3359) -> (11.3993, -48.3289)
  spline S101 degree 2 poles (11.3993, -48.3289) (11.4644, -48.3302) (11.5977, -48.303) (11.6888, -48.2796) knots 0 0 0 1 2 2 2
  spline S102 degree 2 poles (11.6888, -48.2796) (11.9014, -48.2248) (12.2721, -47.9315) (12.4141, -47.7006) knots 0 0 0 1 2 2 2
  line L236 (12.4141, -47.7006) -> (11.8433, -45.4835)
  line L237 (11.8433, -45.4835) -> (12.3698, -45.348)
  line L238 (12.3698, -45.348) -> (13.1743, -48.4728)
  line L239 (13.1743, -48.4728) -> (12.6478, -48.6084)
  line L240 (12.6478, -48.6084) -> (12.528, -48.1427)
  spline S103 degree 2 poles (12.528, -48.1427) (12.3071, -48.473) (11.9324, -48.7926) (11.73, -48.8447) knots 0 0 0 1 2 2 2
  spline S104 degree 2 poles (11.73, -48.8447) (11.649, -48.8655) (11.5663, -48.8796) (11.513, -48.8826) knots 0 0 0 1 2 2 2
  line L241 (11.513, -48.8826) -> (11.3723, -48.3359)
  spline S105 degree 2 poles (8.6058, -46.5571) (8.6612, -46.4964) (8.846, -46.282) (8.9383, -46.2103) knots 0 0 0 1 2 2 2
  spline S106 degree 2 poles (8.9383, -46.2103) (9.0635, -46.1073) (9.311, -45.9763) (9.5503, -45.9288) knots 0 0 0 1 2 2 2
  spline S107 degree 2 poles (9.5503, -45.9288) (9.7451, -45.89) (10.1263, -45.967) (10.2861, -46.0738) knots 0 0 0 1 2 2 2
  spline S108 degree 2 poles (10.2861, -46.0738) (10.4384, -46.1785) (10.6683, -46.5307) (10.7104, -46.7426) knots 0 0 0 1 2 2 2
  spline S109 degree 2 poles (10.7104, -46.7426) (10.7757, -47.0707) (10.5913, -47.5906) (10.317, -47.7837) knots 0 0 0 1 2 2 2
  spline S110 degree 2 poles (10.317, -47.7837) (10.0749, -47.9597) (9.3687, -48.196) (8.9531, -48.3036) knots 0 0 0 1 2 2 2
  line L242 (8.9531, -48.3036) -> (8.9735, -48.4061)
  spline S111 degree 2 poles (8.9735, -48.4061) (9.0102, -48.5906) (9.1685, -48.7972) (9.2839, -48.8418) knots 0 0 0 1 2 2 2
  spline S112 degree 2 poles (9.2839, -48.8418) (9.3994, -48.8863) (9.7014, -48.8689) (9.8587, -48.8376) knots 0 0 0 1 2 2 2
  spline S113 degree 2 poles (9.8587, -48.8376) (10.0432, -48.8009) (10.5204, -48.5923) (10.7489, -48.4368) knots 0 0 0 1 2 2 2
  line L243 (10.7489, -48.4368) -> (10.7796, -48.4306)
  line L244 (10.7796, -48.4306) -> (10.8877, -48.9741)
  spline S114 degree 2 poles (10.8877, -48.9741) (10.7489, -49.0443) (10.219, -49.2562) (9.949, -49.3099) knots 0 0 0 1 2 2 2
  spline S115 degree 2 poles (9.949, -49.3099) (9.6209, -49.3752) (9.1528, -49.3617) (8.9486, -49.2637) knots 0 0 0 1 2 2 2
  spline S116 degree 2 poles (8.9486, -49.2637) (8.7485, -49.1685) (8.4954, -48.7889) (8.4362, -48.4916) knots 0 0 0 1 2 2 2
  line L245 (8.4362, -48.4916) -> (8.006, -46.3282)
  line L246 (8.006, -46.3282) -> (8.5392, -46.2222)
  line L247 (8.5392, -46.2222) -> (8.6058, -46.5571)
  line L248 (8.6942, -47.0014) -> (8.8688, -47.8798)
  spline S117 degree 2 poles (8.8688, -47.8798) (9.0568, -47.8246) (9.6228, -47.6517) (9.7931, -47.561) knots 0 0 0 1 2 2 2
  spline S118 degree 2 poles (9.7931, -47.561) (9.9921, -47.4539) (10.2152, -47.1289) (10.1677, -46.8896) knots 0 0 0 1 2 2 2
  spline S119 degree 2 poles (10.1677, -46.8896) (10.1133, -46.6162) (9.7507, -46.4005) (9.4567, -46.459) knots 0 0 0 1 2 2 2
  spline S120 degree 2 poles (9.4567, -46.459) (9.2072, -46.5086) (8.8399, -46.8055) (8.6942, -47.0014) knots 0 0 0 1 2 2 2
  line L249 (4.7413, -46.7777) -> (5.2804, -46.7082)
  line L250 (5.2804, -46.7082) -> (5.5156, -48.533)
  spline S121 degree 2 poles (5.5156, -48.533) (5.5442, -48.7542) (5.6346, -49.129) (5.7116, -49.235) knots 0 0 0 1 2 2 2
  spline S122 degree 2 poles (5.7116, -49.235) (5.7928, -49.3475) (6.043, -49.4347) (6.2434, -49.4089) knots 0 0 0 1 2 2 2
  spline S123 degree 2 poles (6.2434, -49.4089) (6.4439, -49.383) (6.8413, -49.114) (7.023, -48.9149) knots 0 0 0 1 2 2 2
  line L251 (7.023, -48.9149) -> (6.7146, -46.5233)
  line L252 (6.7146, -46.5233) -> (7.2538, -46.4538)
  line L253 (7.2538, -46.4538) -> (7.6664, -49.6541)
  line L254 (7.6664, -49.6541) -> (7.1272, -49.7236)
  line L255 (7.1272, -49.7236) -> (7.0813, -49.3676)
  spline S124 degree 2 poles (7.0813, -49.3676) (6.8675, -49.6165) (6.4303, -49.9048) (6.1677, -49.9386) knots 0 0 0 1 2 2 2
  spline S125 degree 2 poles (6.1677, -49.9386) (5.6977, -49.9992) (5.0852, -49.4458) (5.009, -48.8548) knots 0 0 0 1 2 2 2
  line L256 (5.009, -48.8548) -> (4.7413, -46.7777)
  spline S126 degree 2 poles (2.5789, -46.8565) (3.3511, -46.8101) (4.2519, -47.6251) (4.3, -48.4251) knots 0 0 0 1 2 2 2
  spline S127 degree 2 poles (4.3, -48.4251) (4.3473, -49.2112) (3.579, -50.193) (2.9146, -50.233) knots 0 0 0 1 2 2 2
  spline S128 degree 2 poles (2.9146, -50.233) (2.6155, -50.251) (2.1424, -50.1049) (1.9609, -49.9308) knots 0 0 0 1 2 2 2
  spline S129 degree 2 poles (1.9609, -49.9308) (1.7759, -49.7569) (1.5595, -49.2358) (1.5363, -48.8497) knots 0 0 0 1 2 2 2
  line L257 (1.5363, -48.8497) -> (1.5185, -48.554)
  line L258 (1.5185, -48.554) -> (3.7481, -48.4199)
  spline S130 degree 2 poles (3.7481, -48.4199) (3.7144, -47.8599) (3.1152, -47.299) (2.6143, -47.3291) knots 0 0 0 1 2 2 2
  spline S131 degree 2 poles (2.6143, -47.3291) (2.4369, -47.3398) (2.0974, -47.4405) (1.962, -47.5115) knots 0 0 0 1 2 2 2
  spline S132 degree 2 poles (1.962, -47.5115) (1.8201, -47.5899) (1.6257, -47.7237) (1.5629, -47.7834) knots 0 0 0 1 2 2 2
  line L259 (1.5629, -47.7834) -> (1.5316, -47.7852)
  line L260 (1.5316, -47.7852) -> (1.4961, -47.1939)
  spline S133 degree 2 poles (1.4961, -47.1939) (1.5877, -47.15) (1.8662, -47.0216) (1.9756, -46.9836) knots 0 0 0 1 2 2 2
  spline S134 degree 2 poles (1.9756, -46.9836) (2.1294, -46.9289) (2.3841, -46.8682) (2.5789, -46.8565) knots 0 0 0 1 2 2 2
  spline S135 degree 2 poles (2.0721, -48.9362) (2.0923, -49.1549) (2.2019, -49.4694) (2.2954, -49.572) knots 0 0 0 1 2 2 2
  spline S136 degree 2 poles (2.2954, -49.572) (2.3966, -49.6881) (2.7, -49.799) (2.9192, -49.7859) knots 0 0 0 1 2 2 2
  spline S137 degree 2 poles (2.9192, -49.7859) (3.1348, -49.7729) (3.4297, -49.626) (3.5474, -49.4932) knots 0 0 0 1 2 2 2
  spline S138 degree 2 poles (3.5474, -49.4932) (3.6614, -49.3572) (3.768, -49.0401) (3.773, -48.8339) knots 0 0 0 1 2 2 2
  line L261 (3.773, -48.8339) -> (2.0721, -48.9362)
  spline S139 degree 2 poles (-3.9923, -48.1824) (-3.9765, -47.8622) (-3.7086, -47.3835) (-3.4988, -47.2333) knots 0 0 0 1 2 2 2
  spline S140 degree 2 poles (-3.4988, -47.2333) (-3.2459, -47.0574) (-2.6847, -46.9247) (-2.2461, -46.9464) knots 0 0 0 1 2 2 2
  line L262 (-2.2461, -46.9464) -> (-1.0141, -47.0072)
  line L263 (-1.0141, -47.0072) -> (-1.2263, -51.302)
  line L264 (-1.2263, -51.302) -> (-2.3643, -51.2458)
  spline S141 degree 2 poles (-2.3643, -51.2458) (-2.8237, -51.2231) (-3.2802, -51.1412) (-3.4834, -51.016) knots 0 0 0 1 2 2 2
  spline S142 degree 2 poles (-3.4834, -51.016) (-3.7105, -50.8827) (-3.9031, -50.472) (-3.8897, -50.2005) knots 0 0 0 1 2 2 2
  spline S143 degree 2 poles (-3.8897, -50.2005) (-3.8747, -49.8977) (-3.5308, -49.4332) (-3.2422, -49.3114) knots 0 0 0 1 2 2 2
  line L265 (-3.2422, -49.3114) -> (-3.2411, -49.2906)
  spline S144 degree 2 poles (-3.2411, -49.2906) (-3.6188, -49.1672) (-4.0126, -48.593) (-3.9923, -48.1824) knots 0 0 0 1 2 2 2
  spline S145 degree 2 poles (-3.396, -48.1874) (-3.408, -48.431) (-3.2843, -48.7511) (-3.0809, -48.8728) knots 0 0 0 1 2 2 2
  spline S146 degree 2 poles (-3.0809, -48.8728) (-2.9486, -48.9491) (-2.6305, -49.0067) (-2.3347, -49.0213) knots 0 0 0 1 2 2 2
  line L266 (-2.3347, -49.0213) -> (-1.6873, -49.0533)
  line L267 (-1.6873, -49.0533) -> (-1.6089, -47.4663)
  line L268 (-1.6089, -47.4663) -> (-2.0718, -47.4434)
  spline S147 degree 2 poles (-2.0718, -47.4434) (-2.4477, -47.4248) (-2.8827, -47.4731) (-3.0553, -47.5762) knots 0 0 0 1 2 2 2
  spline S148 degree 2 poles (-3.0553, -47.5762) (-3.221, -47.6832) (-3.3848, -47.9612) (-3.396, -48.1874) knots 0 0 0 1 2 2 2
  spline S149 degree 2 poles (-3.2906, -50.1499) (-3.2981, -50.303) (-3.2051, -50.5379) (-3.0935, -50.6097) knots 0 0 0 1 2 2 2
  spline S150 degree 2 poles (-3.0935, -50.6097) (-2.9581, -50.6931) (-2.6222, -50.7446) (-2.3194, -50.7595) knots 0 0 0 1 2 2 2
  line L269 (-2.3194, -50.7595) -> (-1.773, -50.7865)
  line L270 (-1.773, -50.7865) -> (-1.7109, -49.5301)
  line L271 (-1.7109, -49.5301) -> (-2.3582, -49.4981)
  spline S151 degree 2 poles (-2.3582, -49.4981) (-2.6262, -49.4849) (-2.883, -49.528) (-3.0231, -49.6083) knots 0 0 0 1 2 2 2
  spline S152 degree 2 poles (-3.0231, -49.6083) (-3.1595, -49.6853) (-3.2806, -49.948) (-3.2906, -50.1499) knots 0 0 0 1 2 2 2
  line L272 (-5, -46.7341) -> (-4.4592, -46.7888)
  line L273 (-4.4592, -46.7888) -> (-4.7839, -49.9991)
  line L274 (-4.7839, -49.9991) -> (-5.3247, -49.9444)
  line L275 (-5.3247, -49.9444) -> (-5, -46.7341)
  line L276 (-5.4169, -50.4745) -> (-4.8032, -50.5366)
  line L277 (-4.8032, -50.5366) -> (-4.86, -51.0982)
  line L278 (-4.86, -51.0982) -> (-5.4737, -51.0361)
  line L279 (-5.4737, -51.0361) -> (-5.4169, -50.4745)
  spline S153 degree 2 poles (-8.6564, -47.8581) (-8.5351, -47.0518) (-7.6276, -46.2898) (-6.9798, -46.3872) knots 0 0 0 1 2 2 2
  spline S154 degree 2 poles (-6.9798, -46.3872) (-6.3148, -46.4873) (-5.6896, -47.5081) (-5.8067, -48.2868) knots 0 0 0 1 2 2 2
  spline S155 degree 2 poles (-5.8067, -48.2868) (-5.927, -49.0863) (-6.8459, -49.8537) (-7.4868, -49.7572) knots 0 0 0 1 2 2 2
  spline S156 degree 2 poles (-7.4868, -49.7572) (-8.1346, -49.6598) (-8.7772, -48.661) (-8.6564, -47.8581) knots 0 0 0 1 2 2 2
  spline S157 degree 2 poles (-8.1017, -47.9416) (-8.195, -48.5619) (-7.8343, -49.2328) (-7.4173, -49.2955) knots 0 0 0 1 2 2 2
  spline S158 degree 2 poles (-7.4173, -49.2955) (-7.0004, -49.3582) (-6.4548, -48.8236) (-6.3615, -48.2034) knots 0 0 0 1 2 2 2
  spline S159 degree 2 poles (-6.3615, -48.2034) (-6.2708, -47.6004) (-6.6323, -46.9117) (-7.0493, -46.849) knots 0 0 0 1 2 2 2
  spline S160 degree 2 poles (-7.0493, -46.849) (-7.4628, -46.7868) (-8.0094, -47.3282) (-8.1017, -47.9416) knots 0 0 0 1 2 2 2
  spline S161 degree 2 poles (-11.971, -47.2289) (-11.796, -46.4397) (-10.8375, -45.6742) (-10.2626, -45.8017) knots 0 0 0 1 2 2 2
  spline S162 degree 2 poles (-10.2626, -45.8017) (-10.0278, -45.8538) (-9.6914, -46.0426) (-9.5292, -46.1963) knots 0 0 0 1 2 2 2
  line L280 (-9.5292, -46.1963) -> (-9.2365, -44.8764)
  line L281 (-9.2365, -44.8764) -> (-8.7058, -44.9941)
  line L282 (-8.7058, -44.9941) -> (-9.6615, -49.3044)
  line L283 (-9.6615, -49.3044) -> (-10.1922, -49.1867)
  line L284 (-10.1922, -49.1867) -> (-10.119, -48.8567)
  spline S163 degree 2 poles (-10.119, -48.8567) (-10.3563, -48.9933) (-10.8922, -49.1243) (-11.1746, -49.0617) knots 0 0 0 1 2 2 2
  spline S164 degree 2 poles (-11.1746, -49.0617) (-11.7155, -48.9417) (-12.131, -47.9502) (-11.971, -47.2289) knots 0 0 0 1 2 2 2
  spline S165 degree 2 poles (-11.4097, -47.2892) (-11.5297, -47.8301) (-11.3181, -48.5016) (-10.9337, -48.5868) knots 0 0 0 1 2 2 2
  spline S166 degree 2 poles (-10.9337, -48.5868) (-10.7091, -48.6366) (-10.2428, -48.5294) (-10.021, -48.4144) knots 0 0 0 1 2 2 2
  line L285 (-10.021, -48.4144) -> (-9.6242, -46.625)
  spline S167 degree 2 poles (-9.6242, -46.625) (-9.8098, -46.4803) (-10.0892, -46.3399) (-10.2797, -46.2976) knots 0 0 0 1 2 2 2
  spline S168 degree 2 poles (-10.2797, -46.2976) (-10.6914, -46.2063) (-11.2815, -46.7108) (-11.4097, -47.2892) knots 0 0 0 1 2 2 2
  line L286 (-14.5763, -44.7009) -> (-14.0551, -44.8553)
  line L287 (-14.0551, -44.8553) -> (-14.5777, -46.6194)
  spline S169 degree 2 poles (-14.5777, -46.6194) (-14.641, -46.8332) (-14.7098, -47.2126) (-14.6823, -47.3407) knots 0 0 0 1 2 2 2
  spline S170 degree 2 poles (-14.6823, -47.3407) (-14.6535, -47.4764) (-14.4599, -47.6573) (-14.2661, -47.7147) knots 0 0 0 1 2 2 2
  spline S171 degree 2 poles (-14.2661, -47.7147) (-14.0724, -47.7721) (-13.6, -47.6867) (-13.3534, -47.5781) knots 0 0 0 1 2 2 2
  line L288 (-13.3534, -47.5781) -> (-12.6685, -45.266)
  line L289 (-12.6685, -45.266) -> (-12.1473, -45.4204)
  line L290 (-12.1473, -45.4204) -> (-13.4231, -49.7271)
  line L291 (-13.4231, -49.7271) -> (-13.9443, -49.5727)
  line L292 (-13.9443, -49.5727) -> (-13.4831, -48.0157)
  spline S172 degree 2 poles (-13.4831, -48.0157) (-13.7793, -48.1569) (-14.2957, -48.2438) (-14.5496, -48.1686) knots 0 0 0 1 2 2 2
  spline S173 degree 2 poles (-14.5496, -48.1686) (-15.004, -48.034) (-15.3404, -47.2802) (-15.1711, -46.7089) knots 0 0 0 1 2 2 2
  line L293 (-15.1711, -46.7089) -> (-14.5763, -44.7009)
  line L294 (-18.7934, -46.6009) -> (-15.6339, -43.0625)
  line L295 (-15.6339, -43.0625) -> (-15.0881, -43.2644)
  line L296 (-15.0881, -43.2644) -> (-16.0974, -44.3252)
  line L297 (-16.0974, -44.3252) -> (-16.0646, -47.6106)
  line L298 (-16.0646, -47.6106) -> (-16.6136, -47.4075)
  line L299 (-16.6136, -47.4075) -> (-16.611, -44.8596)
  line L300 (-16.611, -44.8596) -> (-18.264, -46.7968)
  line L301 (-18.264, -46.7968) -> (-18.7934, -46.6009)
  spline S174 degree 2 poles (-18.8157, -42.9857) (-18.519, -43.116) (-18.0754, -43.5011) (-17.9455, -43.6647) knots 0 0 0 1 2 2 2
  line L302 (-17.9455, -43.6647) -> (-18.1907, -44.223)
  line L303 (-18.1907, -44.223) -> (-18.2162, -44.2118)
  spline S175 degree 2 poles (-18.2162, -44.2118) (-18.2576, -44.1327) (-18.3766, -43.9358) (-18.4908, -43.8058) knots 0 0 0 1 2 2 2
  spline S176 degree 2 poles (-18.4908, -43.8058) (-18.5886, -43.6905) (-18.8557, -43.4667) (-19.0184, -43.3953) knots 0 0 0 1 2 2 2
  spline S177 degree 2 poles (-19.0184, -43.3953) (-19.1365, -43.3434) (-19.4315, -43.2786) (-19.5149, -43.2952) knots 0 0 0 1 2 2 2
  spline S178 degree 2 poles (-19.5149, -43.2952) (-19.634, -43.3152) (-19.7772, -43.416) (-19.8389, -43.5564) knots 0 0 0 1 2 2 2
  spline S179 degree 2 poles (-19.8389, -43.5564) (-19.9159, -43.7319) (-19.8043, -43.9978) (-19.5853, -44.1663) knots 0 0 0 1 2 2 2
  spline S180 degree 2 poles (-19.5853, -44.1663) (-19.4994, -44.2306) (-19.2211, -44.4289) (-19.1057, -44.5215) knots 0 0 0 1 2 2 2
  spline S181 degree 2 poles (-19.1057, -44.5215) (-18.8109, -44.7689) (-18.684, -45.3118) (-18.8114, -45.6021) knots 0 0 0 1 2 2 2
  spline S182 degree 2 poles (-18.8114, -45.6021) (-18.988, -46.0041) (-19.8109, -46.2403) (-20.3087, -46.0217) knots 0 0 0 1 2 2 2
  spline S183 degree 2 poles (-20.3087, -46.0217) (-20.5543, -45.9138) (-20.9988, -45.5741) (-21.1273, -45.4073) knots 0 0 0 1 2 2 2
  line L304 (-21.1273, -45.4073) -> (-20.8933, -44.8745)
  line L305 (-20.8933, -44.8745) -> (-20.8678, -44.8857)
  spline S184 degree 2 poles (-20.8678, -44.8857) (-20.7436, -45.1229) (-20.3549, -45.5029) (-20.1156, -45.608) knots 0 0 0 1 2 2 2
  spline S185 degree 2 poles (-20.1156, -45.608) (-19.8699, -45.7158) (-19.4406, -45.6569) (-19.3496, -45.4496) knots 0 0 0 1 2 2 2
  spline S186 degree 2 poles (-19.3496, -45.4496) (-19.2669, -45.2613) (-19.3881, -44.9912) (-19.5862, -44.8357) knots 0 0 0 1 2 2 2
  spline S187 degree 2 poles (-19.5862, -44.8357) (-19.6821, -44.7593) (-19.9312, -44.5814) (-20.0658, -44.4805) knots 0 0 0 1 2 2 2
  spline S188 degree 2 poles (-20.0658, -44.4805) (-20.3548, -44.2546) (-20.5199, -43.7293) (-20.3756, -43.4006) knots 0 0 0 1 2 2 2
  spline S189 degree 2 poles (-20.3756, -43.4006) (-20.2915, -43.2092) (-19.9931, -42.9368) (-19.7917, -42.8769) knots 0 0 0 1 2 2 2
  spline S190 degree 2 poles (-19.7917, -42.8769) (-19.5779, -42.8147) (-19.1188, -42.8526) (-18.8157, -42.9857) knots 0 0 0 1 2 2 2
  line L306 (-20.9487, -42.0741) -> (-20.4607, -42.3135)
  line L307 (-20.4607, -42.3135) -> (-21.8821, -45.2103)
  line L308 (-21.8821, -45.2103) -> (-22.3702, -44.9708)
  line L309 (-22.3702, -44.9708) -> (-20.9487, -42.0741)
  line L310 (-22.641, -45.4357) -> (-22.0873, -45.7074)
  line L311 (-22.0873, -45.7074) -> (-22.3359, -46.2142)
  line L312 (-22.3359, -46.2142) -> (-22.8896, -45.9425)
  line L313 (-22.8896, -45.9425) -> (-22.641, -45.4357)
  spline S191 degree 2 poles (-22.7545, -41.0421) (-22.4609, -41.2024) (-22.0731, -41.6483) (-21.9989, -41.9269) knots 0 0 0 1 2 2 2
  spline S192 degree 2 poles (-21.9989, -41.9269) (-21.923, -42.2026) (-22.0341, -42.8644) (-22.2378, -43.2376) knots 0 0 0 1 2 2 2
  spline S193 degree 2 poles (-22.2378, -43.2376) (-22.4414, -43.6107) (-22.9374, -44.0467) (-23.2058, -44.1384) knots 0 0 0 1 2 2 2
  spline S194 degree 2 poles (-23.2058, -44.1384) (-23.4759, -44.2332) (-24.0829, -44.1599) (-24.3705, -44.003) knots 0 0 0 1 2 2 2
  spline S195 degree 2 poles (-24.3705, -44.003) (-24.6029, -43.8761) (-24.9655, -43.5075) (-25.087, -43.3301) knots 0 0 0 1 2 2 2
  line L314 (-25.087, -43.3301) -> (-24.7948, -42.7948)
  line L315 (-24.7948, -42.7948) -> (-24.7673, -42.8098)
  spline S196 degree 2 poles (-24.7673, -42.8098) (-24.7387, -42.881) (-24.6397, -43.0779) (-24.5583, -43.1978) knots 0 0 0 1 2 2 2
  spline S197 degree 2 poles (-24.5583, -43.1978) (-24.484, -43.3018) (-24.2566, -43.5252) (-24.1342, -43.592) knots 0 0 0 1 2 2 2
  spline S198 degree 2 poles (-24.1342, -43.592) (-23.7641, -43.794) (-23.009, -43.4796) (-22.7302, -42.9688) knots 0 0 0 1 2 2 2
  spline S199 degree 2 poles (-22.7302, -42.9688) (-22.4581, -42.4702) (-22.587, -41.6734) (-22.9724, -41.4631) knots 0 0 0 1 2 2 2
  spline S200 degree 2 poles (-22.9724, -41.4631) (-23.2049, -41.3362) (-23.7321, -41.2986) (-23.976, -41.36) knots 0 0 0 1 2 2 2
  line L316 (-23.976, -41.36) -> (-24.0036, -41.3449)
  line L317 (-24.0036, -41.3449) -> (-23.7114, -40.8097)
  spline S201 degree 2 poles (-23.7114, -40.8097) (-23.6227, -40.8144) (-23.3569, -40.8365) (-23.2595, -40.8618) knots 0 0 0 1 2 2 2
  spline S202 degree 2 poles (-23.2595, -40.8618) (-23.1171, -40.8919) (-22.9044, -40.9603) (-22.7545, -41.0421) knots 0 0 0 1 2 2 2
  spline S203 degree 2 poles (-24.7461, -39.8677) (-24.471, -40.0389) (-24.0867, -40.4833) (-23.9815, -40.6637) knots 0 0 0 1 2 2 2
  line L318 (-23.9815, -40.6637) -> (-24.3036, -41.1814)
  line L319 (-24.3036, -41.1814) -> (-24.3273, -41.1667)
  spline S204 degree 2 poles (-24.3273, -41.1667) (-24.357, -41.0825) (-24.4468, -40.8707) (-24.5413, -40.7257) knots 0 0 0 1 2 2 2
  spline S205 degree 2 poles (-24.5413, -40.7257) (-24.6217, -40.5977) (-24.8542, -40.3381) (-25.005, -40.2442) knots 0 0 0 1 2 2 2
  spline S206 degree 2 poles (-25.005, -40.2442) (-25.1145, -40.1761) (-25.3973, -40.0699) (-25.4822, -40.0745) knots 0 0 0 1 2 2 2
  spline S207 degree 2 poles (-25.4822, -40.0745) (-25.603, -40.0773) (-25.7591, -40.1567) (-25.8401, -40.2868) knots 0 0 0 1 2 2 2
  spline S208 degree 2 poles (-25.8401, -40.2868) (-25.9414, -40.4495) (-25.8688, -40.7287) (-25.676, -40.9266) knots 0 0 0 1 2 2 2
  spline S209 degree 2 poles (-25.676, -40.9266) (-25.6001, -41.0026) (-25.3529, -41.2385) (-25.2519, -41.3465) knots 0 0 0 1 2 2 2
  spline S210 degree 2 poles (-25.2519, -41.3465) (-24.9953, -41.6334) (-24.947, -42.1888) (-25.1145, -42.458) knots 0 0 0 1 2 2 2
  spline S211 degree 2 poles (-25.1145, -42.458) (-25.3465, -42.8308) (-26.1947, -42.9473) (-26.6562, -42.6601) knots 0 0 0 1 2 2 2
  spline S212 degree 2 poles (-26.6562, -42.6601) (-26.884, -42.5184) (-27.2756, -42.1187) (-27.379, -41.9354) knots 0 0 0 1 2 2 2
  line L320 (-27.379, -41.9354) -> (-27.0715, -41.4413)
  line L321 (-27.0715, -41.4413) -> (-27.0479, -41.456)
  spline S213 degree 2 poles (-27.0479, -41.456) (-26.9587, -41.7085) (-26.6281, -42.14) (-26.4062, -42.2781) knots 0 0 0 1 2 2 2
  spline S214 degree 2 poles (-26.4062, -42.2781) (-26.1784, -42.4198) (-25.7451, -42.4227) (-25.6254, -42.2304) knots 0 0 0 1 2 2 2
  spline S215 degree 2 poles (-25.6254, -42.2304) (-25.5168, -42.0558) (-25.5982, -41.7712) (-25.7722, -41.5891) knots 0 0 0 1 2 2 2
  spline S216 degree 2 poles (-25.7722, -41.5891) (-25.8562, -41.4999) (-26.0775, -41.2883) (-26.1963, -41.1692) knots 0 0 0 1 2 2 2
  spline S217 degree 2 poles (-26.1963, -41.1692) (-26.4502, -40.9045) (-26.5388, -40.361) (-26.3492, -40.0562) knots 0 0 0 1 2 2 2
  spline S218 degree 2 poles (-26.3492, -40.0562) (-26.2387, -39.8787) (-25.9045, -39.6516) (-25.6966, -39.621) knots 0 0 0 1 2 2 2
  spline S219 degree 2 poles (-25.6966, -39.621) (-25.4762, -39.5899) (-25.0272, -39.6928) (-24.7461, -39.8677) knots 0 0 0 1 2 2 2
  line L322 (-31.5343, -37.0872) -> (-30.3924, -37.9914)
  line L323 (-30.3924, -37.9914) -> (-29.4882, -36.8495)
  line L324 (-29.4882, -36.8495) -> (-29.1112, -37.1481)
  line L325 (-29.1112, -37.1481) -> (-30.0154, -38.29)
  line L326 (-30.0154, -38.29) -> (-28.8735, -39.1942)
  line L327 (-28.8735, -39.1942) -> (-29.1612, -39.5575)
  line L328 (-29.1612, -39.5575) -> (-30.3031, -38.6533)
  line L329 (-30.3031, -38.6533) -> (-31.2073, -39.7952)
  line L330 (-31.2073, -39.7952) -> (-31.5843, -39.4967)
  line L331 (-31.5843, -39.4967) -> (-30.6801, -38.3548)
  line L332 (-30.6801, -38.3548) -> (-31.822, -37.4506)
  line L333 (-31.822, -37.4506) -> (-31.5343, -37.0872)
  line L334 (-34.7911, -34.0507) -> (-33.7366, -35.0555)
  line L335 (-33.7366, -35.0555) -> (-32.7318, -34.001)
  line L336 (-32.7318, -34.001) -> (-32.3837, -34.3327)
  line L337 (-32.3837, -34.3327) -> (-33.3885, -35.3872)
  line L338 (-33.3885, -35.3872) -> (-32.3339, -36.392)
  line L339 (-32.3339, -36.392) -> (-32.6536, -36.7275)
  line L340 (-32.6536, -36.7275) -> (-33.7082, -35.7228)
  line L341 (-33.7082, -35.7228) -> (-34.7129, -36.7773)
  line L342 (-34.7129, -36.7773) -> (-35.0611, -36.4456)
  line L343 (-35.0611, -36.4456) -> (-34.0563, -35.391)
  line L344 (-34.0563, -35.391) -> (-35.1108, -34.3863)
  line L345 (-35.1108, -34.3863) -> (-34.7911, -34.0507)
  line L346 (-37.7569, -30.7294) -> (-36.7986, -31.8263)
  line L347 (-36.7986, -31.8263) -> (-35.7016, -30.868)
  line L348 (-35.7016, -30.868) -> (-35.3853, -31.2301)
  line L349 (-35.3853, -31.2301) -> (-36.4822, -32.1884)
  line L350 (-36.4822, -32.1884) -> (-35.5239, -33.2854)
  line L351 (-35.5239, -33.2854) -> (-35.8729, -33.5903)
  line L352 (-35.8729, -33.5903) -> (-36.8312, -32.4933)
  line L353 (-36.8312, -32.4933) -> (-37.9281, -33.4516)
  line L354 (-37.9281, -33.4516) -> (-38.2445, -33.0895)
  line L355 (-38.2445, -33.0895) -> (-37.1476, -32.1312)
  line L356 (-37.1476, -32.1312) -> (-38.1059, -31.0343)
  line L357 (-38.1059, -31.0343) -> (-37.7569, -30.7294)
  line L358 (-40.2132, -24.3987) -> (-39.8978, -24.8753)
  line L359 (-39.8978, -24.8753) -> (-42.9869, -26.9194)
  line L360 (-42.9869, -26.9194) -> (-40.2667, -26.4649)
  line L361 (-40.2667, -26.4649) -> (-40.0744, -26.7555)
  line L362 (-40.0744, -26.7555) -> (-41.562, -29.0727)
  line L363 (-41.562, -29.0727) -> (-38.4729, -27.0287)
  line L364 (-38.4729, -27.0287) -> (-38.1787, -27.4733)
  line L365 (-38.1787, -27.4733) -> (-41.7647, -29.8462)
  line L366 (-41.7647, -29.8462) -> (-42.1955, -29.1952)
  line L367 (-42.1955, -29.1952) -> (-40.7913, -26.9791)
  line L368 (-40.7913, -26.9791) -> (-43.3608, -27.4342)
  line L369 (-43.3608, -27.4342) -> (-43.7992, -26.7716)